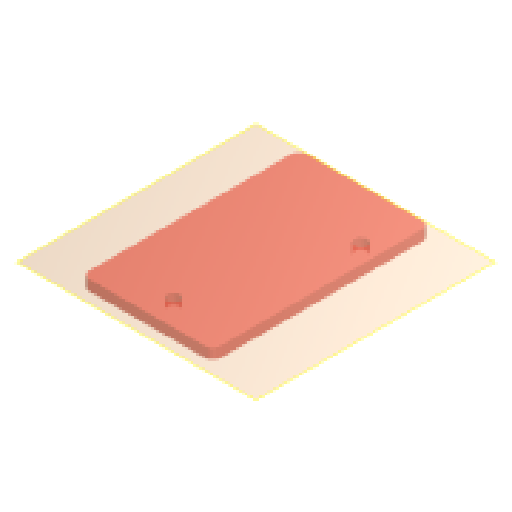
# Autodesk Inventor part: 20_Cube_4_insert_xy_slider
Saved by Autodesk Inventor 2025.1 (Build 291241020, 241B)
## iProperties
Created: 2024-10-07
Part Number: 20_Cube_4_insert_xy_slider
Material: Generic
Document SubType Name: Modeling
Designer: diederichbenedict
Density: 1 g/cm^3
Appearance: Dark Red
Author: diederichbenedict
Autodesk Inventor part; units mm, degrees
ref_plane "YZ Plane" through (0, 0, 0) normal (1, 0, 0) x (0, 1, 0)
ref_plane "XZ Plane" through (0, 0, 0) normal (0, 1, 0) x (-1, 0, 0)
ref_plane "XY Plane" through (0, 0, 0) normal (0, 0, 1) x (1, 0, 0)
ref_plane "Work Plane1" through (0, 0, 0) normal (0, 0, 1) x (1, 0, 0)
sketch "Sketch1" plane through (0, 0, 0) normal (0, 0, 1) x (1, 0, 0)
  arc A0 (1.5114, -4.263) -> (1.1737, -4.342) centre (1.4126, -4.6023) ccw projected
  arc A1 (-11.5885, -9.6282) -> (1.1737, -4.342) centre (-12.45, 10.5) ccw projected
  arc A2 (-11.5885, -9.6282) -> (-11.8831, -9.8112) centre (-11.5734, -9.9812) ccw projected
  arc A3 (-13.0169, -9.8112) -> (-11.8831, -9.8112) centre (-12.45, -9.5) ccw projected
  arc A4 (-13.0169, -9.8112) -> (-13.3115, -9.6282) centre (-13.3266, -9.9812) ccw projected
  arc A5 (-26.0737, -4.342) -> (-13.3115, -9.6282) centre (-12.45, 10.5) ccw projected
  arc A6 (-26.0737, -4.342) -> (-26.4114, -4.263) centre (-26.3126, -4.6023) ccw projected
  arc A7 (-27.213, -3.4614) -> (-26.4114, -4.263) centre (-26.5921, -3.6421) ccw projected
  arc A8 (-27.213, -3.4614) -> (-27.292, -3.1237) centre (-27.5523, -3.3626) ccw projected
  arc A9 (-32.5782, 9.6385) -> (-27.292, -3.1237) centre (-12.45, 10.5) ccw projected
  arc A10 (-32.5782, 9.6385) -> (-32.7612, 9.9331) centre (-32.9312, 9.6234) ccw projected
  arc A11 (-32.7612, 11.0669) -> (-32.7612, 9.9331) centre (-32.45, 10.5) ccw projected
  arc A12 (-32.7612, 11.0669) -> (-32.5782, 11.3615) centre (-32.9312, 11.3766) ccw projected
  arc A13 (-27.292, 24.1237) -> (-32.5782, 11.3615) centre (-12.45, 10.5) ccw projected
  arc A14 (-27.292, 24.1237) -> (-27.213, 24.4614) centre (-27.5523, 24.3626) ccw projected
  arc A15 (-26.4114, 25.263) -> (-27.213, 24.4614) centre (-26.5921, 24.6421) ccw projected
  arc A16 (-26.4114, 25.263) -> (-26.0737, 25.342) centre (-26.3126, 25.6023) ccw projected
  arc A17 (-13.3115, 30.6282) -> (-26.0737, 25.342) centre (-12.45, 10.5) ccw projected
  arc A18 (-13.3115, 30.6282) -> (-13.0169, 30.8112) centre (-13.3266, 30.9812) ccw projected
  arc A19 (-11.8831, 30.8112) -> (-13.0169, 30.8112) centre (-12.45, 30.5) ccw projected
  arc A20 (-11.8831, 30.8112) -> (-11.5885, 30.6282) centre (-11.5734, 30.9812) ccw projected
  arc A21 (1.1737, 25.342) -> (-11.5885, 30.6282) centre (-12.45, 10.5) ccw projected
  arc A22 (1.1737, 25.342) -> (1.5114, 25.263) centre (1.4126, 25.6023) ccw projected
  arc A23 (2.313, 24.4614) -> (1.5114, 25.263) centre (1.6921, 24.6421) ccw projected
  arc A24 (2.313, 24.4614) -> (2.392, 24.1237) centre (2.6523, 24.3626) ccw projected
  arc A25 (7.6782, 11.3615) -> (2.392, 24.1237) centre (-12.45, 10.5) ccw projected
  arc A26 (7.6782, 11.3615) -> (7.8612, 11.0669) centre (8.0313, 11.3766) ccw projected
  arc A27 (7.8612, 9.9331) -> (7.8612, 11.0669) centre (7.55, 10.5) ccw projected
  arc A28 (7.8612, 9.9331) -> (7.6782, 9.6385) centre (8.0313, 9.6234) ccw projected
  arc A29 (2.392, -3.1237) -> (7.6782, 9.6385) centre (-12.45, 10.5) ccw projected
  arc A30 (2.392, -3.1237) -> (2.313, -3.4614) centre (2.6523, -3.3626) ccw projected
  arc A31 (1.5114, -4.263) -> (2.313, -3.4614) centre (1.6921, -3.6421) ccw projected
  arc A32 (-36.6117, 25.3443) -> (-37.35, 24.9048) centre (-36.85, 24.9048) ccw projected
  line L0 (-37.35, 24.9048) -> (-37.35, -3.9048) projected
  arc A33 (-37.35, -3.9048) -> (-36.6117, -4.3443) centre (-36.85, -3.9048) ccw projected
  line L1 (-36.6117, -4.3443) -> (-34.9957, -3.4684) projected
  arc A34 (-34.9957, -4.4161) -> (-34.9957, -3.4684) centre (-34.4238, -3.9422) ccw projected
  line L2 (-34.9957, -4.4161) -> (-37.35, -5.6921) projected
  line L3 (-37.35, -5.6921) -> (-37.35, -6.7071) projected
  arc A35 (-37.35, -6.7071) -> (-36.4964, -7.0607) centre (-36.85, -6.7071) ccw projected
  line L4 (-36.4964, -7.0607) -> (-35.9358, -6.5) projected
  line L5 (-35.9358, -6.5) -> (-33.45, -6.5) projected
  line L6 (-33.45, -6.5) -> (-29.45, -10.5) projected
  line L7 (-29.45, -10.5) -> (-29.3819, -14.4) projected
  line L8 (4.4819, -14.4) -> (-29.3819, -14.4) projected
  line L9 (4.4819, -14.4) -> (4.55, -10.5) projected
  line L10 (8.55, -6.5) -> (4.55, -10.5) projected
  line L11 (11.0358, -6.5) -> (8.55, -6.5) projected
  line L12 (11.5964, -7.0607) -> (11.0358, -6.5) projected
  arc A36 (11.5964, -7.0607) -> (12.45, -6.7071) centre (11.95, -6.7071) ccw projected
  line L13 (12.45, -5.6921) -> (12.45, -6.7071) projected
  line L14 (12.45, -5.6921) -> (10.0957, -4.4161) projected
  arc A37 (10.0957, -3.4684) -> (10.0957, -4.4161) centre (9.5238, -3.9422) ccw projected
  line L15 (10.0957, -3.4684) -> (11.7117, -4.3443) projected
  arc A38 (11.7117, -4.3443) -> (12.45, -3.9048) centre (11.95, -3.9048) ccw projected
  line L16 (12.45, -3.9048) -> (12.45, 24.9048) projected
  arc A39 (12.45, 24.9048) -> (11.7117, 25.3443) centre (11.95, 24.9048) ccw projected
  line L17 (11.7117, 25.3443) -> (10.0957, 24.4684) projected
  arc A40 (10.0957, 25.4161) -> (10.0957, 24.4684) centre (9.5238, 24.9422) ccw projected
  line L18 (10.0957, 25.4161) -> (12.45, 26.6921) projected
  line L19 (12.45, 26.6921) -> (12.45, 27.7071) projected
  arc A41 (12.45, 27.7071) -> (11.5964, 28.0607) centre (11.95, 27.7071) ccw projected
  line L20 (11.5964, 28.0607) -> (11.0358, 27.5) projected
  line L21 (11.0358, 27.5) -> (8.55, 27.5) projected
  line L22 (8.55, 27.5) -> (4.55, 31.5) projected
  line L23 (4.55, 31.5) -> (4.4819, 35.4) projected
  line L24 (-29.3819, 35.4) -> (4.4819, 35.4) projected
  line L25 (-29.3819, 35.4) -> (-29.45, 31.5) projected
  line L26 (-33.45, 27.5) -> (-29.45, 31.5) projected
  line L27 (-35.9358, 27.5) -> (-33.45, 27.5) projected
  line L28 (-36.4964, 28.0607) -> (-35.9358, 27.5) projected
  arc A42 (-36.4964, 28.0607) -> (-37.35, 27.7071) centre (-36.85, 27.7071) ccw projected
  line L29 (-37.35, 27.7071) -> (-37.35, 26.6921) projected
  line L30 (-37.35, 26.6921) -> (-34.9957, 25.4161) projected
  arc A43 (-34.9957, 24.4684) -> (-34.9957, 25.4161) centre (-34.4238, 24.9422) ccw projected
  line L31 (-34.9957, 24.4684) -> (-36.6117, 25.3443) projected
  circle A44 centre (4.05, 27) radius 1.4 projected
  circle A45 centre (4.05, -6) radius 1.4 projected
  circle A46 centre (-28.95, 27) radius 1.4 projected
  circle A47 centre (-28.95, -6) radius 1.4 projected
  line L32 (0.55, -14.5) -> (-25.45, -14.5)
  line L33 (-27.45, -12.5) -> (-27.45, 33.5)
  line L34 (-25.45, 35.5) -> (0.55, 35.5)
  line L35 (2.55, 33.5) -> (2.55, -12.5)
  line L36 (2.55, -14.5) -> (-27.45, 35.5) construction
  line L37 (-27.45, -14.5) -> (2.55, 35.5) construction
  arc A48 (-27.45, -12.5) -> (-25.45, -14.5) centre (-25.45, -12.5) ccw
  arc A49 (0.55, -14.5) -> (2.55, -12.5) centre (0.55, -12.5) ccw
  arc A50 (2.55, 33.5) -> (0.55, 35.5) centre (0.55, 33.5) ccw
  arc A51 (-25.45, 35.5) -> (-27.45, 33.5) centre (-25.45, 33.5) ccw
  circle A52 centre (-1.95, 24) radius 1.4
  circle A53 centre (-12.45, 10.5) radius 12.5
  point P0 (0, 0)
  point P1 (-26.0745, -14.4)
  point P2 (1.1745, -14.4)
  point P3 (1.1745, 35.4)
  point P4 (-26.0745, 35.4)
  dimension "d0" = 30
  dimension "d1" = 50
  dimension "d2" = 2
  dimension "d3" = 2.8
  dimension "d4" = 25
  dimension "d7" = 6
  dimension "d8" = 3
  constraints: 12 end point, 8 point on circle, 8 point on line, 8 tangent, 6 centre point, 3 equal radius, 2 midpoint, 2 parallel, 1 coincident, 1 horizontal, 1 perpendicular
  measures "d0" distance of L36.end L37.end
  measures "d1" distance of L37.start L36.end
  measures "d2" radius of A48
  measures "d3" diameter of A52
  measures "d4" diameter of A53
  measures "d7" horizontal distance of A44.centre A52.centre
  measures "d8" vertical distance of A44.centre A52.centre
extrude "Extrusion1" add sketch "Sketch1" along normal blind 2.4 contours A31 A30 A29 L35 A49 L8 A48 L33 A9 A8 A7 A6 A5 A4 A3 A2 A1 A0 | A0 A1 A2 A3 A4 A5 A6 A7 A8 A9 L33 A13 A14 A15 A16 A17 A18 A19 A20 A21 A22 A23 A24 A25 L35 A29 A30 A31 | A25 A24 A23 A22 A21 A20 A19 A18 A17 A16 A15 A14 A13 L33 A51 L24 A50 L35 | A53
sketch "Sketch2" plane through (0, 0, 2.4) normal (0, 0, 1) x (1, 0, 0)
  arc A0 (-27.45, -12.5) -> (-26.0745, -14.4) centre (-25.45, -12.5) ccw projected
  line L0 (-26.0745, -14.4) -> (1.1745, -14.4) projected
  arc A1 (1.1745, -14.4) -> (2.55, -12.5) centre (0.55, -12.5) ccw projected
  line L1 (2.55, -12.5) -> (2.55, 33.5) projected
  arc A2 (2.55, 33.5) -> (1.1745, 35.4) centre (0.55, 33.5) ccw projected
  line L2 (1.1745, 35.4) -> (-26.0745, 35.4) projected
  arc A3 (-26.0745, 35.4) -> (-27.45, 33.5) centre (-25.45, 33.5) ccw projected
  line L3 (-27.45, 33.5) -> (-27.45, -12.5) projected
  circle A4 centre (-1.95, 24) radius 1.4 projected
  circle A5 centre (-12.45, -8.4) radius 1.4
  point P0 (0, 0)
  point P1 (-12.45, -14.4)
  dimension "d9" = 2.8
  dimension "d10" = 6
  constraints: 1 centre point, 1 midpoint
  measures "d9" diameter of A5
  measures "d10" distance of point (-12.45, -14.4) A5.centre
extrude "Extrusion2" cut sketch "Sketch2" against normal through all contours A5
body "Solid1"
